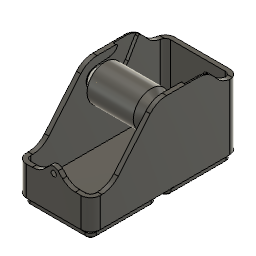
SnapTools-1U-Solder-Wire-Holder (Autodesk Fusion 360 design; units mm, degrees)
Autodesk Fusion 360 part; units mm, degrees
sketch "Sketch1" plane through (0, 0, 0) normal (0, 1, 0) x (1, 0, 0) in component "SnapTools - 1U-Solder-Wire-Holder - Base"
  line L0 (-18.6, -2.4) -> (18.6, -2.4)
  line L1 (18.6, -2.4) -> (18.6, -39.6)
  line L2 (18.6, -39.6) -> (-18.6, -39.6)
  line L3 (-18.6, -39.6) -> (-18.6, -2.4)
  line L4 (-18.6, 2.4) -> (18.6, 2.4)
  line L5 (18.6, 2.4) -> (18.6, 39.6)
  line L6 (18.6, 39.6) -> (-18.6, 39.6)
  line L7 (-18.6, 39.6) -> (-18.6, 2.4)
  line L8 (-18.6, 2.4) -> (18.6, 39.6) construction
  circle A0 centre (-13, 8) radius 3.125
  line L9 (0, 21) -> (18.6, 21) construction
  line L10 (18.6, 2.4) -> (0, 21) construction
  circle A1 centre (13, 8) radius 3.125
  circle A2 centre (13, 34) radius 3.125
  circle A3 centre (-13, 34) radius 3.125
  line L11 (0, 0) -> (34, 0) construction
  circle A4 centre (-13, -34) radius 3.125
  circle A5 centre (-13, -8) radius 3.125
  circle A6 centre (13, -8) radius 3.125
  circle A7 centre (13, -34) radius 3.125
  circle A8 centre (0, 21) radius 5.125
  circle A9 centre (0, -21) radius 5.125
  dimension "d15" = 37.2
  dimension "d16" = 4.8
  dimension "d17" = 18.6
  dimension "d18" = 2.4
  dimension "d19" = 79.2
  dimension "d20" = 39.6
  dimension "d21" = 37.2
  dimension "d25" = 5.6
  dimension "d26" = 6.25
  dimension "d27" = 6.25
  dimension "d28" = 5.6
  dimension "d110" = 10.25
  constraint horizontal L0
  constraint vertical L1
  constraint horizontal L2
  constraint vertical L3
  constraint horizontal L4
  constraint vertical L5
  constraint horizontal L6
  constraint vertical L7
  constraint collinear L1 L5
  constraint collinear L3 L7
  constraint coincident L8 A0.centre
  constraint midpoint L8 L9.start
  constraint midpoint L5 L9.end
  constraint coincident L10 A1.centre
  constraint symmetric A0 L9 A3
  constraint symmetric L9 A1 A2
  constraint coincident L11.start origin
  constraint parallel L4 L11
  constraint symmetric A0 L11 A5
  constraint symmetric A1 L11 A6
  constraint symmetric A2 L11 A7
  constraint symmetric A3 L11 A4
  constraint coincident L9.start L10.end
  constraint symmetric L11 A8 A9
  measures "d15" distance of L1.end L2.end
  measures "d16" distance of L0 L4
  measures "d17" horizontal distance of L11.start L1.end
  measures "d18" vertical distance of L11.start L0.end
  measures "d19" distance of L2 L6
  measures "d20" distance of L11.start L2
  measures "d21" distance of L0 L2
  measures "d25" distance of L4 A0.centre
  measures "d26" diameter of A0
  measures "d27" diameter of A1
  measures "d28" distance of L4 A1.centre
  measures "d110" diameter of A8
extrude "Extrude1" add sketch "Sketch1" along normal blind 2.6 contours L0 L1 L2 L3 | L4 L5 L6 L7 | A0 | A1 | A2 | A3 | A4 | A5 | A6 | A7 | A8 | A9 makes body 1 at (-6.2, 0, 27.2) makes body 2 at (-6.2, 0, -27.2) in component "SnapTools - 1U-Solder-Wire-Holder - Base"
fillet "Fillet3" radius 3.2 8 edges at (18.6, 1.3, 2.4) (-18.6, 1.3, 2.4) (-18.6, 1.3, 39.6) (18.6, 1.3, 39.6) (-18.6, 1.3, -39.6) (-18.6, 1.3, -2.4) (18.6, 1.3, -2.4) (18.6, 1.3, -39.6) on bodies 1 2 in component "SnapTools - 1U-Solder-Wire-Holder - Base"
chamfer "Chamfer4" distance 0.8 angle 45 16 edges at (-18.6, 0, 21) (-17.6627, 0, 3.3373) (0, 0, 2.4) (17.6627, 0, 3.3373) (18.6, 0, 21) (17.6627, 0, 38.6627) (0, 0, 39.6) (-17.6627, 0, 38.6627) (-18.6, 0, -21) (-17.6627, 0, -3.3373) (0, 0, -2.4) (17.6627, 0, -3.3373) (18.6, 0, -21) (17.6627, 0, -38.6627) (0, 0, -39.6) (-17.6627, 0, -38.6627) on bodies 1 2 in component "SnapTools - 1U-Solder-Wire-Holder - Base"
extrude "Extrude7" add 1 faces at (5.1333, 2.6, -14.8) along direction (0, 1, 0) blind 2.15 draft 45 on bodies 2 bodies 2 in component "SnapTools - 1U-Solder-Wire-Holder - Base"
extrude "Extrude8" add 1 faces at (5.1333, 2.6, 14.8) along direction (0, 1, 0) blind 2.15 draft 45 on bodies 1 bodies 1 in component "SnapTools - 1U-Solder-Wire-Holder - Base"
sketch "Sketch6" plane through (0, 4.75, 0) normal (0, 1, 0) x (-1, 0, 0) in component "SnapTools - 1U-Solder-Wire-Holder - Base"
  line L0 (-20.75, -5.6) -> (-20.75, -36.4)
  arc A0 (-20.75, -36.4) -> (-15.4, -41.75) centre (-15.4, -36.4) ccw
  line L1 (-15.4, -41.75) -> (15.4, -41.75)
  arc A1 (15.4, -41.75) -> (20.75, -36.4) centre (15.4, -36.4) ccw
  line L2 (20.75, -36.4) -> (20.75, -5.6)
  arc A2 (20.75, -5.6) -> (15.4, -0.25) centre (15.4, -5.6) ccw
  line L3 (15.4, -0.25) -> (-15.4, -0.25)
  arc A3 (-15.4, -0.25) -> (-20.75, -5.6) centre (-15.4, -5.6) ccw
  line L4 (15.4, 41.75) -> (-15.4, 41.75)
  arc A4 (-15.4, 41.75) -> (-20.75, 36.4) centre (-15.4, 36.4) ccw
  line L5 (-20.75, 36.4) -> (-20.75, 5.6)
  arc A5 (-20.75, 5.6) -> (-15.4, 0.25) centre (-15.4, 5.6) ccw
  line L6 (-15.4, 0.25) -> (15.4, 0.25) construction
  arc A6 (15.4, 0.25) -> (20.75, 5.6) centre (15.4, 5.6) ccw
  line L7 (20.75, 5.6) -> (20.75, 36.4)
  arc A7 (20.75, 36.4) -> (15.4, 41.75) centre (15.4, 36.4) ccw
  line L8 (20.75, -5.6) -> (20.75, 5.6)
  line L9 (-20.75, -5.6) -> (-20.75, 5.6)
  constraint coincident L2.end A2.start
  constraint coincident A6.end L7.start
  constraint coincident L0.start A3.end
  constraint coincident L5.end A5.start
extrude "Extrude10" add sketch "Sketch6" along normal blind 2.25 bodies 1 2 in component "SnapTools - 1U-Solder-Wire-Holder - Base"
extrude "Extrude5" cut sketch "Sketch1" along normal blind 2.25 contours A0 | A1 | A2 | A3 | A4 | A5 | A6 | A7 bodies 1 in component "SnapTools - 1U-Solder-Wire-Holder - Base"
extrude "Extrude6" cut 8 faces at (-12.0499, 2.25, -33.3928) (13.9501, 2.25, -34.6072) (-13.4152, 2.25, -7.4926) (12.6331, 2.25, -7.3237) (13.9124, 2.25, 8.7544) (-13.4152, 2.25, 8.5074) (-12.0499, 2.25, 34.6072) (13.9501, 2.25, 33.3928) along direction (0, 1, 0) blind 1.5 draft -55 on bodies 1 bodies 1 in component "SnapTools - 1U-Solder-Wire-Holder - Base"
sketch "Sketch1 (2)" plane through (0, 7, 0) normal (0, 1, 0) x (-1, 0, 0) in component "SnapTools - 1U-Solder-Wire-Holder - Base"
  arc A0 (-20.75, -36.4) -> (-15.4, -41.75) centre (-15.4, -36.4) ccw
  line L0 (-15.4, -41.75) -> (15.4, -41.75)
  arc A1 (15.4, -41.75) -> (20.75, -36.4) centre (15.4, -36.4) ccw
  line L1 (20.75, -36.4) -> (20.75, 36.4)
  arc A2 (20.75, 36.4) -> (15.4, 41.75) centre (15.4, 36.4) ccw
  line L2 (15.4, 41.75) -> (-15.4, 41.75)
  arc A3 (-15.4, 41.75) -> (-20.75, 36.4) centre (-15.4, 36.4) ccw
  line L3 (-20.75, 36.4) -> (-20.75, -36.4)
  line L4 (-15.4, -39.25) -> (15.4, -39.25)
  arc A4 (15.4, -39.25) -> (18.25, -36.4) centre (15.4, -36.4) ccw
  line L5 (18.25, -36.4) -> (18.25, 36.4)
  arc A5 (18.25, 36.4) -> (15.4, 39.25) centre (15.4, 36.4) ccw
  line L6 (15.4, 39.25) -> (-15.4, 39.25)
  arc A6 (-15.4, 39.25) -> (-18.25, 36.4) centre (-15.4, 36.4) ccw
  line L7 (-18.25, 36.4) -> (-18.25, -36.4)
  arc A7 (-18.25, -36.4) -> (-15.4, -39.25) centre (-15.4, -36.4) ccw
  line L8 (18.024, -25.192) -> (-17.976, -25.192) construction
  line L9 (-17.976, -25.192) -> (-17.976, 13.508) construction
  line L10 (-17.976, 13.508) -> (18.024, 13.508) construction
  line L11 (18.024, 13.508) -> (18.024, -25.192) construction
  dimension "d66" = 36.5
  dimension "d67" = 36
  dimension "d68" = 38.7
  constraint horizontal L8
  constraint vertical L9
  constraint horizontal L10
  constraint vertical L11
  measures "d66" distance of L5 L7
  measures "d67" distance of L8.start L8.end
  measures "d68" distance of L8.start L10.end
extrude "Extrude11" add sketch "Sketch1 (2)" along normal blind 44.35 bodies 1 in component "SnapTools - 1U-Solder-Wire-Holder - Base"
sketch "Sketch2" plane through (-20.75, 0, 0) normal (-1, 0, 0) x (0, 0, 1) in component "SnapTools - 1U-Solder-Wire-Holder - Base"
  line L0 (-36.4, 4.75) -> (-5.6, 4.75)
  line L1 (-5.6, 4.75) -> (5.6, 4.75)
  line L2 (5.6, 4.75) -> (36.4, 4.75)
  line L3 (36.4, 4.75) -> (36.4, 51.35)
  line L4 (36.4, 51.35) -> (-36.4, 51.35)
  line L5 (-36.4, 51.35) -> (-36.4, 4.75)
  line L6 (-36.4, 7) -> (-39.25, 7)
  line L7 (-36.4, 7) -> (36.4, 7)
  line L8 (39.25, 7) -> (36.4, 7)
  line L9 (39.25, 7) -> (36.4, 7)
  line L10 (36.4, 7) -> (-36.4, 7)
  line L11 (-36.4, 7) -> (-39.25, 7)
  circle A0 centre (0, 41.35) radius 5 construction
  circle A1 centre (0, 41.35) radius 19.35 construction
  line L12 (41.75, 4.75) -> (41.75, 51.35)
  line L13 (41.75, 21.3966) -> (29.797, 21.3966)
  line L14 (29.797, 21.3966) -> (4.6631, 51.35)
  line L15 (-24.2442, 51.35) -> (-32.6352, 41.35)
  line L16 (-41.75, 4.75) -> (-41.75, 51.35)
  line L17 (-32.6352, 41.35) -> (-41.75, 41.35)
  line L18 (0, 7) -> (0, 51.35) construction
  line L19 (-24.2442, 51.35) -> (-41.75, 51.35)
  line L20 (4.6631, 51.35) -> (41.75, 51.35)
  dimension "d71" = 10
  dimension "d72" = 34.35
  dimension "d73" = 38.7
  dimension "d74" = 130
  dimension "d75" = 10
  dimension "d76" = 130
  dimension "d77" = 10
  dimension "d78" = 25
  constraint concentric A0 A1
  constraint coincident L12 L13.start
  constraint perpendicular L3 L13
  constraint coincident L4 L14.end
  constraint coincident L4 L15.start
  constraint coincident L16 L17.end
  constraint perpendicular L16 L17
  constraint midpoint L10 L18.start
  constraint midpoint L4 L18.end
  constraint coincident A0.centre L18
  constraint coincident L16.end L19.end
  constraint coincident L12.end L20.end
  measures "d71" diameter of A0
  measures "d72" distance of L10 A0.centre
  measures "d73" diameter of A1
  measures "d74" angle of L13 L14
  measures "d75" distance of A0.centre L14
  measures "d76" angle of L15 L17
  measures "d77" distance of L4 L17
  measures "d78" distance of A0.centre L15
extrude "Extrude12" cut sketch "Sketch2" against normal through all contours L5 L16 L17 L19 | L4 L5 L15 L17 L19 | L3 L4 L13 L14 L20 | L3 L12 L13 L20 bodies 1 in component "SnapTools - 1U-Solder-Wire-Holder - Base"
sketch "Sketch3" plane through (18.25, 0, 0) normal (-1, 0, 0) x (0, 0, 1) in component "SnapTools - 1U-Solder-Wire-Holder - Base"
  line L0 (-32.6352, 41.35) -> (-36.4, 41.35)
  line L1 (-36.4, 41.35) -> (-36.4, 7)
  line L2 (-36.4, 7) -> (36.4, 7)
  line L3 (36.4, 7) -> (36.4, 21.3966)
  line L4 (36.4, 21.3966) -> (29.797, 21.3966)
  line L5 (29.797, 21.3966) -> (4.6631, 51.35)
  line L6 (4.6631, 51.35) -> (-24.2442, 51.35)
  line L7 (-24.2442, 51.35) -> (-32.6352, 41.35)
  line L8 (0, 7) -> (0, 51.35) construction
  circle A0 centre (0, 41.35) radius 5 construction
  circle A1 centre (0, 41.35) radius 5.25
  line L9 (0.4576, 46.58) -> (-8.2225, 47.3394)
  line L10 (-12.1169, 49.8204) -> (-13, 51.35)
  line L11 (-0.4576, 36.12) -> (-14.5828, 37.3558)
  line L12 (-18.4772, 39.8368) -> (-25.1244, 51.35)
  arc A2 (-12.1169, 49.8204) -> (-8.2225, 47.3394) centre (-7.7868, 52.3204) ccw
  arc A3 (-18.4772, 39.8368) -> (-14.5828, 37.3558) centre (-14.147, 42.3368) ccw
  dimension "d80" = 10
  dimension "d81" = 34.35
  dimension "d82" = 0.25
  dimension "d83" = 10.5
  dimension "d84" = 5
  dimension "d85" = 60
  dimension "d86" = 5
  dimension "d87" = 5
  dimension "d88" = 13
  constraint midpoint L2 L8.start
  constraint coincident L6 L8.end
  constraint perpendicular L6 L8
  constraint coincident L8 A0.centre
  constraint coincident A1 L9.start
  constraint coincident L6 L10.end
  constraint coincident A1 L11.start
  constraint coincident L6 L12.end
  constraint parallel L10 L12
  constraint tangent A1 L9
  constraint tangent A1 L11
  constraint parallel L9 L11
  constraint tangent L10 A2
  constraint tangent L9 A2
  constraint tangent L12 A3
  constraint tangent L11 A3
  measures "d80" diameter of A0
  measures "d81" distance of L8.start A0.centre
  measures "d83" distance of L10 L12
  measures "d84" angle of L6 L9
  measures "d85" angle of L6 L10
  measures "d86" radius of A2
  measures "d87" radius of A3
  measures "d88" horizontal distance of A0.centre L10.end
extrude "Extrude13" cut sketch "Sketch3" against normal up to surface (1.7 mm away) contours L6 L7 A1 L9 L10 L11 L12 A2 A3 | A1 bodies 1 in component "SnapTools - 1U-Solder-Wire-Holder - Base"
extrude "Extrude14" cut 1 faces at (19.95, 40.2717, -7.7543) along direction (-1, 0, 0) up to surface (1.7 mm away) from surface at 38.2 on bodies 1 bodies 1 in component "SnapTools - 1U-Solder-Wire-Holder - Base"
sketch "Sketch7" plane through (0, 0, 41.75) normal (0, 0, 1) x (1, 0, 0) in component "SnapTools - 1U-Solder-Wire-Holder - Base"
  line L0 (15.4, 21.3966) -> (-15.4, 21.3966)
  line L1 (-15.4, 21.3966) -> (-15.4, 4.75)
  line L2 (-15.4, 4.75) -> (15.4, 4.75)
  line L3 (15.4, 4.75) -> (15.4, 21.3966)
  circle A0 centre (0, 24.3966) radius 1.5
  circle A1 centre (0, 24.3966) radius 3.5
  line L4 (0, 21.3966) -> (0, 31) construction
  line L5 (-2.4749, 26.8715) -> (-7.9497, 21.3966)
  line L6 (2.4749, 26.8715) -> (7.9497, 21.3966)
  dimension "d95" = 3
  dimension "d96" = 2
  dimension "d97" = 3
  dimension "d98" = 45
  dimension "d99" = 45
  constraint midpoint L0 L4.start
  constraint perpendicular L0 L4
  constraint coincident A0.centre L4
  constraint coincident A1 L5.start
  constraint coincident L0 L5.end
  constraint coincident A1 L6.start
  constraint coincident L0 L6.end
  constraint tangent A1 L6
  constraint tangent A1 L5
  measures "d95" diameter of A0
  measures "d97" distance of A0.centre L4.start
  measures "d98" angle of L0 L5
  measures "d99" angle of L0 L6
extrude "Extrude15" add sketch "Sketch7" against normal up to surface (2.5 mm away) contours L0 A1 L6 | L0 A1 | L0 A1 L5 picked at (-0.0374, 21.898) bodies 1 in component "SnapTools - 1U-Solder-Wire-Holder - Base"
fillet "Fillet4" radius 10 2 edges at (-7.9497, 21.3966, 40.5) (7.9497, 21.3966, 40.5) on bodies 1 in component "SnapTools - 1U-Solder-Wire-Holder - Base"
fillet "Fillet5" radius 12 8 edges at (19.5, 21.3966, 29.797) (19.5, 51.35, 4.6631) (-19.5, 51.35, 4.6631) (-19.5, 21.3966, 29.797) (-20.35, 51.35, -24.2442) (-19.5, 41.35, -32.6352) (20.35, 51.35, -24.2442) (19.5, 41.35, -32.6352) on bodies 1 in component "SnapTools - 1U-Solder-Wire-Holder - Base"
fillet "Fillet6" radius 0.8 4 edges at (19.1, 49.9326, -24.306) (19.1, 51.35, -13) (-19.1, 49.9326, -24.306) (-19.1, 51.35, -13) on bodies 1 in component "SnapTools - 1U-Solder-Wire-Holder - Base"
extrude "Extrude16" cut sketch "Sketch1" along normal blind 5.25 contours A8 | A9 bodies 1 in component "SnapTools - 1U-Solder-Wire-Holder - Base"
extrude "Extrude17" cut 2 faces at (0.6241, 5.25, -22.3687) (0.6241, 5.25, 19.6313) along direction (0, 1, 0) blind 0.8 draft -60 on bodies 1 bodies 1 in component "SnapTools - 1U-Solder-Wire-Holder - Base"
sketch "Sketch1 (3)" plane through (19.95, 0, 0) normal (-1, 0, 0) x (0, 0, 1) in component "SnapTools - 1U-Solder-Wire-Holder - Axle 10mm"
  arc A0 (-18.6485, 51.35) -> (-25.0233, 49.5167) centre (-18.6485, 39.35) ccw
  arc A1 (-23.9055, 49.2389) -> (-25.0233, 49.5167) centre (-24.5983, 48.8389) ccw
  line L0 (-23.9055, 49.2389) -> (-18.4772, 39.8368)
  arc A2 (-18.4772, 39.8368) -> (-14.5828, 37.3558) centre (-14.147, 42.3368) ccw
  line L1 (-14.5828, 37.3558) -> (-0.4576, 36.12)
  arc A3 (-0.4576, 36.12) -> (0.4576, 46.58) centre (0, 41.35) ccw
  line L2 (0.4576, 46.58) -> (-8.2225, 47.3394)
  arc A4 (-12.1169, 49.8204) -> (-8.2225, 47.3394) centre (-7.7868, 52.3204) ccw
  line L3 (-12.1169, 49.8204) -> (-12.3072, 50.15)
  arc A5 (-11.6144, 51.35) -> (-12.3072, 50.15) centre (-11.6144, 50.55) ccw
  line L4 (-11.6144, 51.35) -> (-18.6485, 51.35)
  circle A6 centre (0, 41.35) radius 5
  dimension "d115" = 10
  constraint concentric A3 A6
  measures "d115" diameter of A6
extrude "Extrude1'" add sketch "Sketch1 (3)" along normal up to surface (39.65 mm away) from surface at 0.125 separate body contours A6 makes body 3 in component "SnapTools - 1U-Solder-Wire-Holder - Axle 10mm"
sketch "Sketch1 (4)" plane through (19.95, 0, 0) normal (-1, 0, 0) x (0, 0, 1) in component "SnapTools - 1U-Solder-Wire-Holder - Axle 20mm"
  arc A0 (-18.6485, 51.35) -> (-25.0233, 49.5167) centre (-18.6485, 39.35) ccw
  arc A1 (-23.9055, 49.2389) -> (-25.0233, 49.5167) centre (-24.5983, 48.8389) ccw
  line L0 (-23.9055, 49.2389) -> (-18.4772, 39.8368)
  arc A2 (-18.4772, 39.8368) -> (-14.5828, 37.3558) centre (-14.147, 42.3368) ccw
  line L1 (-14.5828, 37.3558) -> (-0.4576, 36.12)
  arc A3 (-0.4576, 36.12) -> (0.4576, 46.58) centre (0, 41.35) ccw
  line L2 (0.4576, 46.58) -> (-8.2225, 47.3394)
  arc A4 (-12.1169, 49.8204) -> (-8.2225, 47.3394) centre (-7.7868, 52.3204) ccw
  line L3 (-12.1169, 49.8204) -> (-12.3072, 50.15)
  arc A5 (-11.6144, 51.35) -> (-12.3072, 50.15) centre (-11.6144, 50.55) ccw
  line L4 (-11.6144, 51.35) -> (-18.6485, 51.35)
  circle A6 centre (0, 41.35) radius 5
  circle A7 centre (0, 41.35) radius 10
  dimension "d115_1" = 10
  dimension "d119" = 20
  constraint concentric A3 A6
  constraint concentric A6 A7
  measures "d115_1" diameter of A6
  measures "d119" diameter of A7
extrude "Extrude1''" add sketch "Sketch1 (4)" along normal up to surface (39.65 mm away) from surface at 0.125 separate body contours A6 makes body 4 in component "SnapTools - 1U-Solder-Wire-Holder - Axle 20mm"
extrude "Extrude2" add sketch "Sketch1 (4)" along normal up to surface (36 mm away) from surface at 1.95 contours L1 A3 L2 A7 | L1 A3 L2 A7 bodies 4 in component "SnapTools - 1U-Solder-Wire-Holder - Axle 20mm"
chamfer "Chamfer1" distance 5 angle 45 2 edges at (-18, 37.7338, -9.3233) (18, 44.9662, -9.3233) on bodies 4 in component "SnapTools - 1U-Solder-Wire-Holder - Axle 20mm"
sketch "Sketch1 (5)" plane through (19.95, 0, 0) normal (-1, 0, 0) x (0, 0, 1) in component "SnapTools - 1U-Solder-Wire-Holder - Axle Parametric"
  arc A0 (-18.6485, 51.35) -> (-25.0233, 49.5167) centre (-18.6485, 39.35) ccw
  arc A1 (-23.9055, 49.2389) -> (-25.0233, 49.5167) centre (-24.5983, 48.8389) ccw
  line L0 (-23.9055, 49.2389) -> (-18.4772, 39.8368)
  arc A2 (-18.4772, 39.8368) -> (-14.5828, 37.3558) centre (-14.147, 42.3368) ccw
  line L1 (-14.5828, 37.3558) -> (-0.4576, 36.12)
  arc A3 (-0.4576, 36.12) -> (0.4576, 46.58) centre (0, 41.35) ccw
  line L2 (0.4576, 46.58) -> (-8.2225, 47.3394)
  arc A4 (-12.1169, 49.8204) -> (-8.2225, 47.3394) centre (-7.7868, 52.3204) ccw
  line L3 (-12.1169, 49.8204) -> (-12.3072, 50.15)
  arc A5 (-11.6144, 51.35) -> (-12.3072, 50.15) centre (-11.6144, 50.55) ccw
  line L4 (-11.6144, 51.35) -> (-18.6485, 51.35)
  circle A6 centre (0, 41.35) radius 5
  circle A7 centre (0, 41.35) radius 7.5
  dimension "d115_1_1" = 10
  dimension "d119_1" = 15
  constraint concentric A3 A6
  constraint concentric A6 A7
  measures "d115_1_1" diameter of A6
  measures "d119_1" diameter of A7
extrude "Extrude1'''" add sketch "Sketch1 (5)" along normal up to surface (39.65 mm away) from surface at 0.125 separate body contours A6 makes body 5 in component "SnapTools - 1U-Solder-Wire-Holder - Axle Parametric"
extrude "Extrude2'" add sketch "Sketch1 (5)" along normal up to surface (36 mm away) from surface at 1.95 contours L1 A3 L2 A7 | L1 A3 L2 A7 bodies 5 in component "SnapTools - 1U-Solder-Wire-Holder - Axle Parametric"
chamfer "Chamfer1'" distance 2.5 angle 45 2 edges at (-18, 38.6379, -6.9925) (18, 44.0621, -6.9925) on bodies 5 in component "SnapTools - 1U-Solder-Wire-Holder - Axle Parametric"
component "SnapTools - 1U-Solder-Wire-Holder - Base" placed x (1, 0, 0) y (0, 1, 0) z (0, 0, 1) at (0, 0, 0)
component "SnapTools - 1U-Solder-Wire-Holder - Axle 10mm" placed x (1, 0, 0) y (0, 1, 0) z (0, 0, 1) at (0, 0, 0)
component "SnapTools - 1U-Solder-Wire-Holder - Axle 20mm" placed x (1, 0, 0) y (0, 1, 0) z (0, 0, 1) at (0, 0, 0)
component "SnapTools - 1U-Solder-Wire-Holder - Axle Parametric" placed x (1, 0, 0) y (0, 1, 0) z (0, 0, 1) at (0, 0, 0)
equation "printer_offset = 0.25 mm"
equation "solder_spool_width = 36 mm"
equation "solder_spool_diameter = 38.7 mm"
equation "solder_spool_center_hole_diameter = 20 mm"
equation "holder_axle_diameter = 10 mm"
equation "holder_width = 41.5 mm" comment "gridfinity width"
equation "holder_length = 83.5 mm"
equation "holder_solder_spool_bottom_spacing = 15 mm"
equation "holder_axle_slot_angle = 5 deg"
equation "holder_axle_depth = 10 mm"
equation "gridfinity_bottom_chamfer = 0.8 mm"
equation "gridfinity_top_chamfer = 2.15 mm"
equation "gridfinity_chamfer_offset = 0.25 mm"
equation "gridfinity_chamfer_spacing = 1.8 mm"
equation "d15 = holder_width - ( 2 * gridfinity_top_chamfer )"
equation "d16 = 2 * ( gridfinity_top_chamfer + gridfinity_chamfer_offset )"
equation "d17 = d15 / 2"
equation "d18 = d16 / 2"
equation "d19 = holder_length - ( 2 * gridfinity_top_chamfer )"
equation "d20 = d19 / 2"
equation "gridfinity_magnet_hole_size = 6 mm"
equation "gridfinity_magnet_hole_depth = 2 mm"
equation "gridfinity_distance_from_side = gridfinity_bottom_chamfer + 4.8 mm"
equation "d25 = gridfinity_distance_from_side"
equation "d26 = gridfinity_magnet_hole_size + printer_offset"
equation "d27 = d26"
equation "d28 = d25"
equation "d29 = gridfinity_bottom_chamfer + gridfinity_chamfer_spacing"
equation "gridfinity_1u = 7 mm"
equation "d44 = gridfinity_magnet_hole_depth + printer_offset"
equation "gridfinity_top_fillet_radius = 7.5 mm"
equation "gridfinity_bottom_fillet_radius = 3.2 mm"
equation "d54 = gridfinity_top_chamfer"
equation "d56 = gridfinity_top_chamfer"
equation "d61 = gridfinity_bottom_fillet_radius"
equation "d62 = gridfinity_bottom_chamfer"
equation "d63 = gridfinity_1u - gridfinity_bottom_chamfer - gridfinity_chamfer_spacing - gridfinity_top_chamfer"
equation "d66 = solder_spool_width + 2 * printer_offset"
equation "d67 = solder_spool_width"
equation "d68 = solder_spool_diameter"
equation "d69 = solder_spool_diameter / 2 + holder_solder_spool_bottom_spacing + holder_axle_depth"
equation "d71 = holder_axle_diameter"
equation "d72 = solder_spool_diameter / 2 + holder_solder_spool_bottom_spacing"
equation "d73 = solder_spool_diameter"
equation "d80 = holder_axle_diameter"
equation "d81 = solder_spool_diameter / 2 + holder_solder_spool_bottom_spacing"
equation "d82 = printer_offset"
equation "d83 = holder_axle_diameter + 2 * printer_offset"
equation "d84 = holder_axle_slot_angle"
equation "d86 = holder_axle_diameter / 2"
equation "d87 = holder_axle_diameter / 2"
equation "d88 = holder_axle_slot_length"
equation "holder_axle_slot_length = 13 mm"
equation "snaptool_magnet_diameter = 10 mm"
equation "snaptool_magnet_depth = 5 mm"
equation "d110 = snaptool_magnet_diameter + printer_offset"
equation "d111 = snaptool_magnet_depth + printer_offset"
equation "d115 = holder_axle_diameter"
equation "d116 = printer_offset / 2"
equation "d117 = printer_offset / 2"
equation "d115_1 = holder_axle_diameter"
equation "d116_1 = printer_offset / 2"
equation "d117_1 = printer_offset / 2"
equation "d120 = printer_offset"
equation "d121 = printer_offset"
equation "d115_1_1 = holder_axle_diameter"
equation "d116_1_1 = printer_offset / 2"
equation "d117_1_1 = printer_offset / 2"
equation "d119_1 = holder_axle_parametric_size"
equation "d120_1 = printer_offset"
equation "d121_1 = printer_offset"
equation "d123_1 = ( holder_axle_parametric_size - holder_axle_diameter ) / 2"
equation "holder_axle_parametric_size = 15 mm"
named bodies: "SnapTools - 1U-Solder-Wire-Holder - Base", "SnapTools - 1U-Solder-Wire-Holder - Axle 10mm", "SnapTools - 1U-Solder-Wire-Holder - Axle 20mm", "SnapTools - 1U-Solder-Wire-Holder - Axle Parametric"
